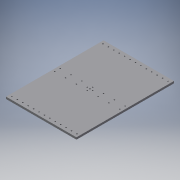
# Autodesk Inventor part: KrackenPlate1
Saved by Autodesk Inventor 2016 (Build 200138000, 138)
## iProperties
Created: 2015-09-06
Part Number: KrackenPlate1
Material: Generic
Document SubType Name: Modeling
Designer: Tim
Density: 1 g/cm^3
Appearance: Default
Author: Tim
Autodesk Inventor part; units mm, degrees
ref_plane "YZ Plane" through (0, 0, 0) normal (1, 0, 0) x (0, 1, 0)
ref_plane "XZ Plane" through (0, 0, 0) normal (0, 1, 0) x (-1, 0, 0)
ref_plane "XY Plane" through (0, 0, 0) normal (0, 0, 1) x (1, 0, 0)
sketch "Sketch1" plane through (0, 0, 0) normal (0, 0, 1) x (1, 0, 0)
  line L0 (104, -144) -> (-104, -144)
  line L1 (-104, -144) -> (-104, 144)
  line L2 (-104, 144) -> (104, 144)
  line L3 (104, 144) -> (104, -144)
  line L4 (104, -144) -> (-104, 144) construction
  line L5 (-104, -144) -> (104, 144) construction
  circle A0 centre (96, 134.4) radius 1.85
  circle A1 centre (80, 134.4) radius 1.85
  circle A2 centre (64, 134.4) radius 1.85
  circle A3 centre (48, 134.4) radius 1.85
  circle A4 centre (32, 134.4) radius 1.85
  circle A5 centre (16, 134.4) radius 1.85
  circle A6 centre (0, 134.4) radius 1.85
  circle A7 centre (-16, 134.4) radius 1.85
  circle A8 centre (-32, 134.4) radius 1.85
  circle A9 centre (-48, 134.4) radius 1.85
  circle A10 centre (-64, 134.4) radius 1.85
  circle A11 centre (-80, 134.4) radius 1.85
  circle A12 centre (-96, 134.4) radius 1.85
  circle A13 centre (48, -134.4) radius 1.85
  circle A14 centre (64, -134.4) radius 1.85
  circle A15 centre (32, -134.4) radius 1.85
  circle A16 centre (16, -134.4) radius 1.85
  circle A17 centre (80, -134.4) radius 1.85
  circle A18 centre (96, -134.4) radius 1.85
  circle A19 centre (0, -134.4) radius 1.85
  circle A20 centre (-16, -134.4) radius 1.85
  circle A21 centre (-32, -134.4) radius 1.85
  circle A22 centre (-48, -134.4) radius 1.85
  circle A23 centre (-80, -134.4) radius 1.85
  circle A24 centre (-96, -134.4) radius 1.85
  line L6 (104, 144) -> (-104, -144) construction
  line L7 (-104, 144) -> (104, -144) construction
  circle A25 centre (-64, -134.4) radius 1.85
  circle A26 centre (0, 0) radius 1.85
  circle A27 centre (-8, 0) radius 1.85 projected
  circle A28 centre (0, -8) radius 1.85 projected
  circle A29 centre (8, 0) radius 1.85 projected
  circle A30 centre (0, 8) radius 1.85 projected
  circle A31 centre (-96, 8) radius 1.85 projected
  circle A32 centre (-96, -8) radius 1.85 projected
  circle A33 centre (96, 8) radius 1.85 projected
  circle A34 centre (96, -8) radius 1.85 projected
  circle A35 centre (64, -8) radius 1.85 projected
  circle A36 centre (64, 8) radius 1.85 projected
  circle A37 centre (32, -8) radius 1.85 projected
  circle A38 centre (32, 8) radius 1.85 projected
  circle A39 centre (-32, -8) radius 1.85 projected
  circle A40 centre (-32, 8) radius 1.85 projected
  circle A41 centre (-64, -8) radius 1.85 projected
  circle A42 centre (-64, 8) radius 1.85 projected
  circle A43 centre (-96, 120) radius 1.85 projected
  circle A44 centre (-96, 104) radius 1.85 projected
  circle A45 centre (-96, 88) radius 1.85 projected
  circle A46 centre (-96, 56) radius 1.85 projected
  circle A47 centre (-96, 40) radius 1.85 projected
  circle A48 centre (-96, 24) radius 1.85 projected
  circle A49 centre (-64, 24) radius 1.85 projected
  circle A50 centre (-64, 56) radius 1.85 projected
  circle A51 centre (-64, 40) radius 1.85 projected
  circle A52 centre (-64, 88) radius 1.85 projected
  circle A53 centre (-64, 72) radius 1.85 projected
  circle A54 centre (-64, 120) radius 1.85 projected
  circle A55 centre (-64, 104) radius 1.85 projected
  circle A56 centre (-32, 120) radius 1.85 projected
  circle A57 centre (-32, 104) radius 1.85 projected
  circle A58 centre (-32, 88) radius 1.85 projected
  circle A59 centre (-32, 72) radius 1.85 projected
  circle A60 centre (0, 88) radius 1.85 projected
  circle A61 centre (0, 104) radius 1.85 projected
  circle A62 centre (0, 120) radius 1.85 projected
  circle A63 centre (32, 120) radius 1.85 projected
  circle A64 centre (32, 104) radius 1.85 projected
  circle A65 centre (64, 120) radius 1.85 projected
  circle A66 centre (64, 104) radius 1.85 projected
  circle A67 centre (64, 88) radius 1.85 projected
  circle A68 centre (32, 88) radius 1.85 projected
  circle A69 centre (32, 72) radius 1.85 projected
  circle A70 centre (64, 72) radius 1.85 projected
  circle A71 centre (0, 72) radius 1.85 projected
  circle A72 centre (-32, 56) radius 1.85 projected
  circle A73 centre (-32, 40) radius 1.85 projected
  circle A74 centre (0, 56) radius 1.85 projected
  circle A75 centre (0, 40) radius 1.85 projected
  circle A76 centre (32, 56) radius 1.85 projected
  circle A77 centre (32, 40) radius 1.85 projected
  circle A78 centre (64, 56) radius 1.85 projected
  circle A79 centre (64, 40) radius 1.85 projected
  circle A80 centre (64, 24) radius 1.85 projected
  circle A81 centre (32, 24) radius 1.85 projected
  circle A82 centre (0, 24) radius 1.85 projected
  circle A83 centre (-32, 24) radius 1.85 projected
  circle A84 centre (-96, 72) radius 1.85 projected
  circle A85 centre (64, -24) radius 1.85 projected
  circle A86 centre (64, -40) radius 1.85 projected
  circle A87 centre (32, -24) radius 1.85 projected
  circle A88 centre (32, -40) radius 1.85 projected
  circle A89 centre (32, -56) radius 1.85 projected
  circle A90 centre (64, -56) radius 1.85 projected
  circle A91 centre (64, -72) radius 1.85 projected
  circle A92 centre (32, -72) radius 1.85 projected
  circle A93 centre (0, -40) radius 1.85 projected
  circle A94 centre (0, -24) radius 1.85 projected
  circle A95 centre (0, -56) radius 1.85 projected
  circle A96 centre (0, -72) radius 1.85 projected
  circle A97 centre (-32, -24) radius 1.85 projected
  circle A98 centre (-64, -24) radius 1.85 projected
  circle A99 centre (-96, -24) radius 1.85 projected
  circle A100 centre (-96, -40) radius 1.85 projected
  circle A101 centre (-64, -40) radius 1.85 projected
  circle A102 centre (-32, -40) radius 1.85 projected
  circle A103 centre (-32, -56) radius 1.85 projected
  circle A104 centre (-64, -56) radius 1.85 projected
  circle A105 centre (-96, -56) radius 1.85 projected
  circle A106 centre (-96, -72) radius 1.85 projected
  circle A107 centre (-64, -72) radius 1.85 projected
  circle A108 centre (-32, -72) radius 1.85 projected
  circle A109 centre (-32, -88) radius 1.85 projected
  circle A110 centre (0, -88) radius 1.85 projected
  circle A111 centre (32, -88) radius 1.85 projected
  circle A112 centre (64, -88) radius 1.85 projected
  circle A113 centre (64, -104) radius 1.85 projected
  circle A114 centre (32, -104) radius 1.85 projected
  circle A115 centre (0, -104) radius 1.85 projected
  circle A116 centre (-32, -104) radius 1.85 projected
  circle A117 centre (-64, -104) radius 1.85 projected
  circle A118 centre (-64, -88) radius 1.85 projected
  circle A119 centre (-96, -88) radius 1.85 projected
  circle A120 centre (-96, -104) radius 1.85 projected
  circle A121 centre (-96, -120) radius 1.85 projected
  circle A122 centre (-64, -120) radius 1.85 projected
  circle A123 centre (-32, -120) radius 1.85 projected
  circle A124 centre (0, -120) radius 1.85 projected
  circle A125 centre (32, -120) radius 1.85 projected
  circle A126 centre (64, -120) radius 1.85 projected
  point P0 (0, 0)
  point P1 (0, 0)
  dimension "d0" = 208
  dimension "d1" = 288
  dimension "d4" = 3.7
  constraints: 16 end point, 4 midpoint, 2 parallel, 1 centre point, 1 coincident, 1 horizontal, 1 perpendicular
  measures "d0" distance of L2.start L2.end
  measures "d1" distance of L2.end L3.end
  measures "d4" diameter of A26
extrude "Extrusion4" add sketch "Sketch1" against normal blind 6
body "Solid4"
